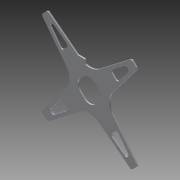
# Autodesk Inventor part: 6061 Bed no holes
Saved by Autodesk Inventor 2014 (Build 180170000, 170)
## iProperties
Created: 2016-05-10
Part Number: 6061 Bed no holes
Material: Aluminum 6061
Document SubType Name: Modeling
Designer: 101767
Density: 2.71 g/cm^3
Appearance: Aluminum - Flat
Mass: 1521.5 g
Surface Area: 1910.74 cm^2
Volume: 561.441 cm^3
Author: 101767
Autodesk Inventor part; units mm, degrees
ref_plane "YZ Plane" through (0, 0, 0) normal (1, 0, 0) x (0, 1, 0)
ref_plane "XZ Plane" through (0, 0, 0) normal (0, 1, 0) x (-1, 0, 0)
ref_plane "XY Plane" through (0, 0, 0) normal (0, 0, 1) x (1, 0, 0)
sketch "Plate" plane through (0, 0, 0) normal (0, 0, 1) x (1, 0, 0)
  line L0 (-200, -200) -> (200, -200) construction
  line L1 (200, -200) -> (200, 200) construction
  line L2 (200, 200) -> (-200, 200) construction
  line L3 (-200, 200) -> (-200, -200) construction
  line L4 (-200, -200) -> (200, 200) construction
  line L5 (200, -200) -> (-200, 200) construction
  line L6 (0, 0) -> (0, 420.657) construction
  line L7 (0, 0) -> (461.6465, 0) construction
  line L8 (0, 202) -> (202, 202) construction
  line L9 (202, 202) -> (202, 0) construction
  line L10 (74.8189, 0) -> (251.7605, 230.5948) construction
  line L11 (254.8388, 145.1612) -> (158.001, 241.999) construction
  line L12 (252.9755, 175.3088) -> (179.3809, 248.9034) construction
  line L13 (74.8189, 0) -> (228.2843, 200)
  line L14 (200, 200) -> (231.4665, 231.4665) construction
  line L15 (228.2843, 200) -> (214.1421, 214.1421)
  line L16 (200, 228.2843) -> (214.1421, 214.1421)
  line L17 (200, 228.2843) -> (0, 74.8189)
  line L18 (-74.8189, 0) -> (-228.2843, 200)
  line L19 (-228.2843, 200) -> (-214.1421, 214.1421)
  line L20 (-200, 228.2843) -> (-214.1421, 214.1421)
  line L21 (-200, 228.2843) -> (0, 74.8189)
  line L22 (74.8189, 0) -> (228.2843, -200)
  line L23 (228.2843, -200) -> (214.1421, -214.1421)
  line L24 (200, -228.2843) -> (214.1421, -214.1421)
  line L25 (200, -228.2843) -> (0, -74.8189)
  line L26 (-200, -228.2843) -> (0, -74.8189)
  line L27 (-200, -228.2843) -> (-214.1421, -214.1421)
  line L28 (-228.2843, -200) -> (-214.1421, -214.1421)
  line L29 (-74.8189, 0) -> (-228.2843, -200)
  dimension "d136" = 10
  dimension "d12" = 200
  dimension "d79" = 200
  dimension "d80" = 2
  dimension "d81" = 2
  dimension "d83" = 20
  dimension "d84" = 7.5
  dimension "d85" = 20
  dimension "d86" = 7.5
  constraints: 60 end point, 12 symmetric about line, 9 point on line, 5 parallel, 5 perpendicular, 2 midpoint, 1 horizontal
  measures "d12" distance between parallel lines of L7 L2
  measures "d79" distance from line of L1.end L6
  measures "d80" distance between parallel lines of L2 L8
  measures "d81" distance between parallel lines of L1 L9
  measures "d83" distance between parallel lines of L11 L12
  measures "d84" angle of L10 L4
  measures "d85" distance from line of L14 L13.end
  measures "d86" angle of L4 L17
extrude "Base" add sketch "Plate" along normal blind 6.35
sketch "Sketch3" plane through (0, 0, 0) normal (0, 0, 1) x (1, 0, 0)
  line L0 (-70.7107, 0) -> (0, 70.7107)
  line L1 (0, 70.7107) -> (70.7107, 0)
  line L2 (70.7107, 0) -> (0, -70.7107)
  line L3 (0, -70.7107) -> (-70.7107, 0)
  line L4 (-70.7107, 0) -> (70.7107, 0) construction
  line L5 (0, 70.7107) -> (0, -70.7107) construction
  point P0 (0, 0)
  dimension "d76" = 90
  dimension "d77" = 100
  constraints: 12 end point, 2 midpoint, 2 parallel, 1 perpendicular, 1 vertical
  measures "d76" angle of L4 L5
  measures "d77" distance of L0.end L1.end
extrude "Center hole" cut sketch "Sketch3" along normal through all
fillet "Fillet2" radius 75 4 edges at (0, 74.8189, 3.175) (-74.8189, 0, 3.175) (0, -74.8189, 3.175) (74.8189, 0, 3.175)
fillet "Fillet3" radius 35 4 edges at (-70.7107, 0, 3.175) (0, 70.7107, 3.175) (70.7107, 0, 3.175) (0, -70.7107, 3.175)
fillet "Fillet4" radius 10 8 edges at (200, 228.2843, 3.175) (228.2843, 200, 3.175) (228.2843, -200, 3.175) (200, -228.2843, 3.175) (-200, -228.2843, 3.175) (-228.2843, -200, 3.175) (-200, 228.2843, 3.175) (-228.2843, 200, 3.175)
sketch "Sketch17" plane through (0, 0, 0) normal (0, 0, 1) x (1, 0, 0)
  line L0 (-200, -200) -> (200, 200) construction
  line L1 (254.8388, 145.1612) -> (158.001, 241.999) construction
  line L2 (182.3223, 182.3223) -> (174.6892, 189.9555)
  line L3 (174.6892, 189.9555) -> (98.6702, 131.6241)
  line L4 (98.6702, 131.6241) -> (115.1472, 115.1472)
  line L5 (193.0425, 222.9456) -> (45.6571, 109.8528) construction
  line L6 (182.3223, 182.3223) -> (189.9555, 174.6892)
  line L7 (189.9555, 174.6892) -> (131.6241, 98.6702)
  line L8 (131.6241, 98.6702) -> (115.1472, 115.1472)
  point P0 (0, 0)
  dimension "d133" = 15
  dimension "d134" = 25
  dimension "d135" = 95
  constraints: 12 end point, 2 parallel, 2 point on line, 2 symmetric about line, 1 perpendicular
  measures "d133" distance between parallel lines of L5 L3
  measures "d134" distance between parallel lines of L2 L1
  measures "d135" distance between parallel lines of L2 L4
extrude "Extrusion4" cut sketch "Sketch17" along normal through all
fillet "Fillet5" radius 10 4 edges at (174.6892, 189.9555, 3.175) (189.9555, 174.6892, 3.175) (131.6241, 98.6702, 3.175) (98.6702, 131.6241, 3.175)
pattern_circular "Circular Pattern2" count 4 over 360 about axis through (0, 0, -10) along (0, 0, 1) of "Extrusion4", "Fillet5"
sketch "Sketch18" plane through (0, 0, 0) normal (0, 0, 1) x (1, 0, 0)
  arc A0 (-45.6571, 109.8528) -> (45.6571, 109.8528) centre (0, 169.3543) ccw construction
  line L0 (-20, 97.0701) -> (-20, 117.5)
  line L1 (-20, 117.5) -> (-55.6231, 117.5)
  line L2 (-69.5, 100.125) -> (-72.5, 100.125) projected
  arc A1 (-69.5, 92.875) -> (-69.5, 98.125) centre (-69.5, 95.5) ccw construction
  line L3 (-45.6571, 109.8528) -> (-193.0425, 222.9456) construction
  line L4 (-55.6231, 117.5) -> (-45.6571, 109.8528)
  arc A2 (-45.6571, 109.8528) -> (-20, 97.0701) centre (0, 169.3543) ccw
  point P0 (0, 0)
  dimension "d144" = 20
  dimension "d146" = 22
  constraints: 6 end point, 3 point on circle, 1 centre point, 1 collinear, 1 concentric, 1 parallel, 1 perpendicular, 1 point on line, 1 tangent, 1 vertical
  measures "d144" distance from line of L0 point (0, 0)
  measures "d146" distance from line of L1 A1.centre
extrude "Limit nub" add sketch "Sketch18" along normal up to surface (6.35 mm away)
fillet "Fillet6" radius 5 3 edges at (-55.6231, 117.5, 3.175) (-20, 97.0701, 3.175) (-20, 117.5, 3.175)
body "Solid1"
